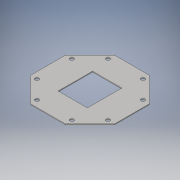
# Autodesk Inventor part: Layer
Saved by Autodesk Inventor 2016 (Build 200138000, 138)
## iProperties
Created: 2019-03-13
Part Number: Layer
Material: Generic
Document SubType Name: Modeling
Designer: isaac
Density: 1 g/cm^3
Appearance: Default
Author: isaac
Autodesk Inventor part; units mm, degrees
ref_plane "YZ Plane" through (0, 0, 0) normal (1, 0, 0) x (0, 1, 0)
ref_plane "XZ Plane" through (0, 0, 0) normal (0, 1, 0) x (-1, 0, 0)
ref_plane "XY Plane" through (0, 0, 0) normal (0, 0, 1) x (1, 0, 0)
sketch "Sketch1" plane through (0, 0, 0) normal (0, 1, 0) x (-1, 0, 0)
  circle A0 centre (0, 0) radius 88.9
  line L0 (0, 0) -> (121.8821, 50.4852)
  line L1 (0, 0) -> (0, 134.8176)
  line L2 (82.1329, 34.0206) -> (82.1329, -34.0206)
  line L3 (82.1329, -34.0206) -> (34.0206, -82.1329)
  line L4 (34.0206, -82.1329) -> (-34.0206, -82.1329)
  line L5 (-34.0206, -82.1329) -> (-82.1329, -34.0206)
  line L6 (-82.1329, -34.0206) -> (-82.1329, 34.0206)
  line L7 (-82.1329, 34.0206) -> (-34.0206, 82.1329)
  line L8 (-34.0206, 82.1329) -> (34.0206, 82.1329)
  line L9 (34.0206, 82.1329) -> (82.1329, 34.0206)
  dimension "d0" = 177.8
  dimension "d1" = 67.5
  dimension "d2" = 164.2658
  constraints: 20 end point, 2 coincident, 1 point on line, 1 vertical, 20 other
  measures "d1" angle of L0 L1
  measures "d2" distance between parallel lines of L4 L8
extrude "Extrusion1" add sketch "Sketch1" along normal blind 1.5875 contours L2 L3 L4 L5 L6 L7 L8 L1 L0 | L0 L1 L8 L9
sketch "Sketch2" plane through (0, 1.5875, 0) normal (0, 1, 0) x (1, 0, 0)
  line L0 (28.575, -33.655) -> (-28.575, -33.655)
  line L1 (-28.575, -33.655) -> (-28.575, 33.655)
  line L2 (-28.575, 33.655) -> (28.575, 33.655)
  line L3 (28.575, 33.655) -> (28.575, -33.655)
  line L4 (28.575, -33.655) -> (-28.575, 33.655) construction
  line L5 (-28.575, -33.655) -> (28.575, 33.655) construction
  point P0 (0, 0)
  dimension "d5" = 57.15
  dimension "d6" = 67.31
  constraints: 12 end point, 2 midpoint, 2 parallel, 1 horizontal, 1 perpendicular
  measures "d5" distance of L1.end L2.end
  measures "d6" distance of L0.end L1.end
extrude "Extrusion2" cut sketch "Sketch2" against normal through all
sketch "Sketch3" plane through (0, 1.5875, 0) normal (0, 1, 0) x (1, 0, 0)
  circle A0 centre (-69.4329, -34.0206) radius 3.6195
  line L0 (-82.1329, 34.0206) -> (-82.1329, -34.0206) projected
  line L1 (-91.914, 0) -> (-48.5333, 0)
  circle A1 centre (-69.4329, 34.0206) radius 3.6195
  circle A2 centre (-34.0206, -69.4329) radius 3.6195
  circle A3 centre (34.0206, -69.4329) radius 3.6195
  circle A4 centre (69.4329, -34.0206) radius 3.6195
  circle A5 centre (69.4329, 34.0206) radius 3.6195
  circle A6 centre (34.0206, 69.4329) radius 3.6195
  circle A7 centre (-34.0206, 69.4329) radius 3.6195
  point P0 (0, 0)
  dimension "d9" = 7.239
  dimension "d10" = 12.7
  dimension "d11" = 0
  dimension "d14" = 360
  constraints: 8 centre point, 2 end point, 1 horizontal, 1 symmetric about line, 18 other
  measures "d9" diameter of A0
  measures "d10" distance from line of A0.centre L0
  measures "d11" vertical distance of A0.centre L0.end
extrude "Extrusion3" cut sketch "Sketch3" against normal through all
body "Solid1"
